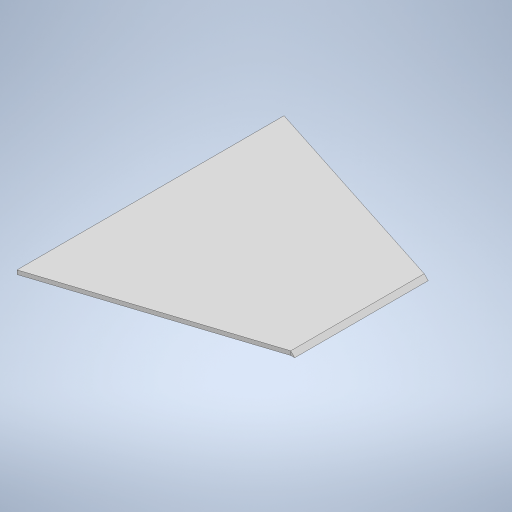
# Autodesk Inventor part: FLU-BackPlateRS3
Saved by Autodesk Inventor 2024.3 (Build 283343000, 343)
## iProperties
Created: 2025-06-13
Part Number: FLU-BackPlateRS3
Material: Generic
Document SubType Name: Modeling
Designer: ajclo
Density: 1 g/cm^3
Appearance: Default
Author: ajclo
Autodesk Inventor part; units mm, degrees
ref_plane "YZ Plane" through (0, 0, 0) normal (1, 0, 0) x (0, 1, 0)
ref_plane "XZ Plane" through (0, 0, 0) normal (0, 1, 0) x (-1, 0, 0)
ref_plane "XY Plane" through (0, 0, 0) normal (0, 0, 1) x (1, 0, 0)
sketch "Sketch1" plane through (0, 0, 0) normal (0, 1, 0) x (-1, 0, 0)
  line L0 (-77.5, 100) -> (77.5, 100)
  line L1 (77.5, 100) -> (77.5, -100)
  line L2 (77.5, -100) -> (-77.5, -100)
  line L3 (-77.5, -100) -> (-77.5, 100)
  line L4 (-77.5, 100) -> (77.5, -100) construction
  line L5 (77.5, 100) -> (-77.5, -100) construction
  line L6 (77.5, 100) -> (-77.5, 50)
  line L7 (-77.5, -50) -> (77.5, -100)
  point P0 (0, 0)
  dimension "d0" = 155
  dimension "d1" = 200
  dimension "d2" = 50
  dimension "d3" = 50
  constraints: 16 end point, 2 midpoint, 2 parallel, 2 point on line, 1 horizontal, 1 perpendicular
  measures "d0" distance of L1.end L2.end
  measures "d1" distance of L0.end L1.end
  measures "d2" distance of L0.start L6.end
  measures "d3" distance of L2.end L7.start
extrude "Extrusion1" add sketch "Sketch1" along normal blind 3 contours L1 L7 L3 L6
sketch "Sketch2" plane through (0, 0, 0) normal (0, 0, 1) x (1, 0, 0)
  line L0 (-77.5, 3) -> (77.5, 3) projected
  line L1 (77.5, 3) -> (80.5, 0)
  line L2 (80.5, 0) -> (77.2748, 0)
  line L3 (-77.5, 0) -> (77.5, 0) projected
  line L4 (77.5, 3) -> (77.5, 0)
  point P0 (0, 0)
  dimension "d6" = 45
  constraints: 6 end point, 1 collinear, 1 parallel, 1 vertical
  measures "d6" angle of L2 L1
extrude "Extrusion2" add sketch "Sketch2" along normal mid plane 100
body "Solid1"
